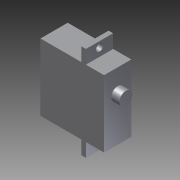
# Autodesk Inventor part: GWS servo micro MG
Saved by Autodesk Inventor 2012 (Build 160160000, 160)
## iProperties
Created: 2013-01-07
Part Number: GWS servo micro MG
Material: Default
Document SubType Name: Modeling
Designer: Irwan Haryanto
Density: 1 g/cm^3
Author: Irwan Haryanto
Autodesk Inventor part; units mm, degrees
ref_plane "YZ Plane" through (0, 0, 0) normal (1, 0, 0) x (0, 1, 0)
ref_plane "XZ Plane" through (0, 0, 0) normal (0, 1, 0) x (-1, 0, 0)
ref_plane "XY Plane" through (0, 0, 0) normal (0, 0, 1) x (1, 0, 0)
sketch "Sketch1" plane through (0, 0, 0) normal (0, 0, 1) x (1, 0, 0)
  line L0 (-4.6523, 10.5287) -> (7.3477, 10.5287)
  line L1 (7.3477, 10.5287) -> (7.3477, -18.9713)
  line L2 (7.3477, -18.9713) -> (-4.6523, -18.9713)
  line L3 (-4.6523, -18.9713) -> (-4.6523, 10.5287)
  line L4 (-4.6523, 10.5287) -> (-4.6523, 16.5287)
  line L5 (-4.6523, 16.5287) -> (7.3477, 16.5287)
  line L6 (7.3477, 16.5287) -> (7.3477, 10.5287)
  line L7 (-4.6523, -18.9713) -> (-4.6523, -24.9713)
  line L8 (-4.6523, -24.9713) -> (7.3477, -24.9713)
  line L9 (7.3477, -24.9713) -> (7.3477, -18.9713)
  circle A0 centre (1.3477, 14.0287) radius 1.5
  circle A1 centre (1.3477, -22.4713) radius 1.5
  point P0 (0, 0)
  dimension "d0" = 12
  dimension "d1" = 29.5
  dimension "d2" = 6
  dimension "d3" = 6
  dimension "d4" = 3
  dimension "d5" = 3
  dimension "d23" = 2.5
  dimension "d24" = 2.5
  dimension "d25" = 3.5
  dimension "d26" = 6
  dimension "d27" = 6
  constraints: 20 end point, 5 parallel, 3 perpendicular, 2 centre point, 1 collinear, 1 horizontal
  measures "d0" distance of L0.start L0.end
  measures "d1" distance of L0.end L1.end
  measures "d2" distance of L0.start L4.end
  measures "d3" distance of L2.end L7.end
  measures "d4" diameter of A0
  measures "d5" diameter of A1
  measures "d23" distance from line of A0.centre L5
  measures "d24" distance from line of L8 A1.centre
  measures "d25" distance from line of L0 A0.centre
  measures "d26" distance from line of A0.centre L4
  measures "d27" distance from line of A1.centre L7
extrude "Extrusion1" add sketch "Sketch1" against normal blind 20 contours L0 L1 L2 L3
extrude "Extrusion2" add sketch "Sketch1" against normal blind 2 contours L4 L5 L6 L0 | L2 L9 L8 L7
extrude "Extrusion3" add sketch "Sketch1" along normal blind 8 contours L0 L1 L2 L3
sketch "Sketch3" plane through (0, 0, 8) normal (0, 0, 1) x (1, 0, 0)
  line L0 (-4.6523, 10.5287) -> (7.3477, 10.5287) projected
  circle A0 centre (1.3477, 0.5287) radius 2.85
  line L1 (-4.6523, -18.9713) -> (-4.6523, 10.5287) projected
  point P0 (0, 0)
  dimension "d18" = 5.7
  dimension "d19" = 10
  dimension "d28" = 6
  constraints: 1 centre point
  measures "d18" diameter of A0
  measures "d19" distance from line of L0 A0.centre
  measures "d28" distance from line of L1 A0.centre
extrude "Extrusion5" add sketch "Sketch3" along normal blind 3.6
body "Solid1"
